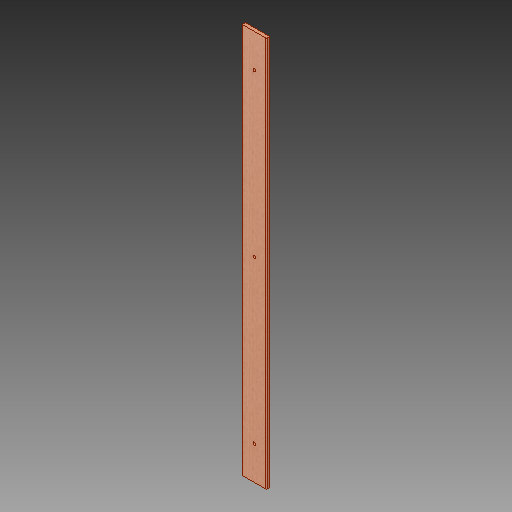
# Autodesk Inventor part: doga_long1
Saved by Autodesk Inventor 2019 (Build 230136000, 136)
## iProperties
Created: 2019-02-23
Part Number: doga_long1
Material: Wood (Oak)
Document SubType Name: Modeling
Designer: gaincarlo
Density: 0.76 g/cm^3
Appearance: White Oak - Natural Medium Gloss
Author: gaincarlo
Autodesk Inventor part; units mm, degrees
ref_plane "YZ Plane" through (0, 0, 0) normal (1, 0, 0) x (0, 1, 0)
ref_plane "XZ Plane" through (0, 0, 0) normal (0, 1, 0) x (-1, 0, 0)
ref_plane "XY Plane" through (0, 0, 0) normal (0, 0, 1) x (1, 0, 0)
ref_plane "Work Plane1" through (0, 0, 0) normal (0, 0, 1) x (1, 0, 0)
sketch "Sketch1" plane through (0, 0, 0) normal (0, 0, 1) x (1, 0, 0)
  line L0 (-45, -725) -> (45, -725)
  line L1 (45, -725) -> (45, 725)
  line L2 (45, 725) -> (-45, 725)
  line L3 (-45, 725) -> (-45, -725)
  line L4 (-385, 0) -> (385, 0) projected
  line L5 (0, -725) -> (0, 725) construction
  circle A0 centre (0, 0) radius 5
  circle A1 centre (0, -600) radius 5
  circle A2 centre (0, 600) radius 5
  circle A3 centre (240, -0.5) radius 5 construction
  circle A4 centre (120, -0.5) radius 5 construction
  circle A5 centre (-120, -0.5) radius 5 construction
  circle A6 centre (-240, -0.5) radius 5 construction
  circle A7 centre (0, -0.5) radius 5 construction
  line L6 (-275, -23) -> (275, -23) construction
  line L7 (275, 23) -> (275, -23) construction
  line L8 (275, 23) -> (-275, 23) construction
  line L9 (-275, -23) -> (-275, 23) construction
  point P0 (0, 0)
  point P1 (-45, 0)
  dimension "d0" = 90
  dimension "d1" = 1450
  dimension "d2" = 10
  dimension "d3" = 10
  dimension "d4" = 10
  dimension "d5" = 600
  dimension "d6" = 600
  constraints: 18 end point, 8 centre point, 4 midpoint, 4 point on line, 3 horizontal, 2 parallel, 2 vertical, 1 perpendicular, 14 other
  measures "d0" distance of L2.end L1.end
  measures "d1" distance of L1.end L0.end
  measures "d2" diameter of A0
  measures "d3" diameter of A1
  measures "d4" diameter of A2
  measures "d5" distance from line of L4 A1.centre
  measures "d6" distance from line of A2.centre L4
extrude "Extrusion1" add sketch "Sketch1" along normal blind 12 contours L3 L4 A0 L1 L0 | L3 L2 L1 L4 A0
fillet "Fillet1" radius 2 6 edges at (-45, -362.5, 12) (-45, 362.5, 12) (-45, -362.5, 0) (-45, 362.5, 0) (45, 0, 12) (45, 0, 0)
body "Solid1"
